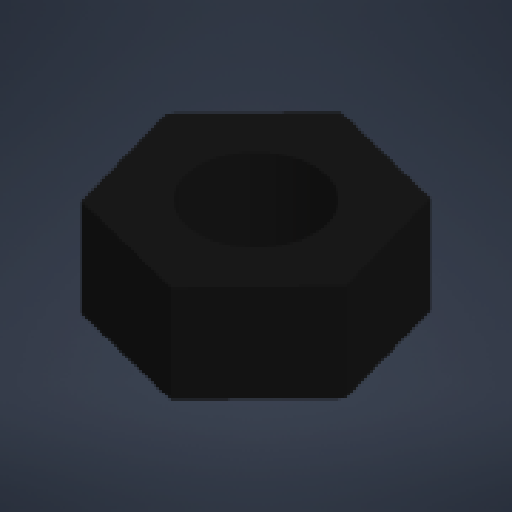
# Autodesk Inventor part: nut
Saved by Autodesk Inventor 2026.2 (Build 302298000, 298)
## iProperties
Created: 2026-01-27
Part Number: nut
Material: Generic
Document SubType Name: Modeling
Designer: test
Density: 1 g/cm^3
Appearance: Default
Author: test
Autodesk Inventor part; units mm, degrees
ref_plane "YZ Plane" through (0, 0, 0) normal (1, 0, 0) x (0, 1, 0)
ref_plane "XZ Plane" through (0, 0, 0) normal (0, 1, 0) x (-1, 0, 0)
ref_plane "XY Plane" through (0, 0, 0) normal (0, 0, 1) x (1, 0, 0)
sketch "Sketch1" plane through (0, 0, 0) normal (0, 1, 0) x (-1, 0, 0)
  line L0 (3.079, -0.7765) -> (0.8671, -3.0547)
  line L1 (0.8671, -3.0547) -> (-2.2119, -2.2783)
  line L2 (-2.2119, -2.2783) -> (-3.079, 0.7765)
  line L3 (-3.079, 0.7765) -> (-0.8671, 3.0547)
  line L4 (-0.8671, 3.0547) -> (2.2119, 2.2783)
  line L5 (2.2119, 2.2783) -> (3.079, -0.7765)
  circle A0 centre (0, 0) radius 1.5
  dimension "d0" = 5.5
  dimension "d1" = 3
  constraints: 12 end point, 2 coincident, 1 centre point, 13 other
  measures "d0" distance between parallel lines of L2 L5
  measures "d1" diameter of A0
extrude "Extrusion1" add sketch "Sketch1" along normal blind 2.5
body "Solid1"
